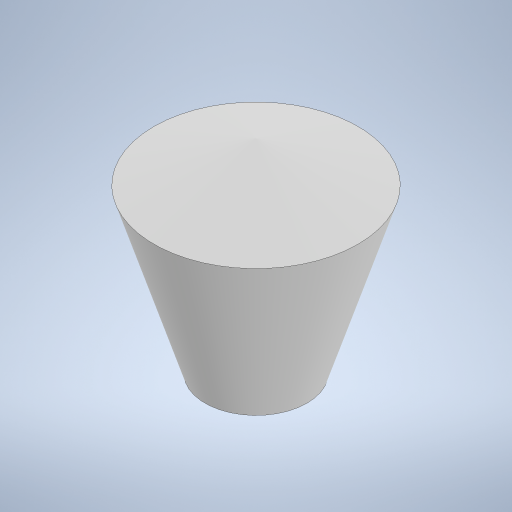
# Autodesk Inventor part: comp
Saved by Autodesk Inventor 2024 (Build 280153000, 153)
## iProperties
Created: 2024-01-16
Part Number: comp
Material: Generic
Document SubType Name: Modeling
Designer: Sorin
Density: 1 g/cm^3
Appearance: Default
Author: Sorin
Autodesk Inventor part; units mm, degrees
ref_plane "YZ Plane" through (0, 0, 0) normal (1, 0, 0) x (0, 1, 0)
ref_plane "XZ Plane" through (0, 0, 0) normal (0, 1, 0) x (-1, 0, 0)
ref_plane "XY Plane" through (0, 0, 0) normal (0, 0, 1) x (1, 0, 0)
sketch "Sketch1" plane through (0, 0, 0) normal (0, 0, 1) x (1, 0, 0)
  line L0 (0, 0) -> (0, 8)
  line L1 (0, 8) -> (1, 8)
  line L2 (1, 8) -> (1, 20)
  line L3 (1, 20) -> (-9, 16)
  line L4 (-4, 0) -> (0, 0)
  line L5 (-9, 16) -> (-4, 0)
  point P0 (-2, 0)
  dimension "d0" = 8
  dimension "d1" = 1
  dimension "d2" = 20
  dimension "d3" = 4
  dimension "d6" = 10
  dimension "d8" = 4
  constraints: 12 end point, 2 perpendicular, 1 midpoint, 1 parallel, 1 vertical
  measures "d0" distance of L0.start L0.end
  measures "d1" distance between parallel lines of L2 L0
  measures "d2" vertical distance of L2.end point (-2, 0)
  measures "d3" distance of L4.start L0.start
  measures "d6" horizontal distance of L2.end L3.end
  measures "d8" vertical distance of L2.end L3.end
revolve "Revolution1" add sketch "Sketch1" angle 360 about axis through (1, 8, 0) along (0, 1, 0)
body "Solid1"
